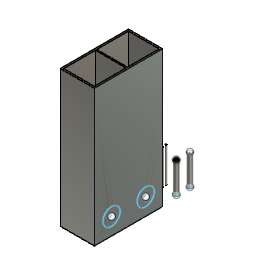
feeder v1 (Autodesk Fusion 360 design; units mm, degrees)
Autodesk Fusion 360 part; units mm, degrees
sketch "Sketch1" plane through (0, 0, 0) normal (0, 0, 1) x (1, 0, 0)
  line L0 (25, 50) -> (-25, 50)
  line L1 (-25, 50) -> (-25, -50)
  line L2 (-25, -50) -> (25, -50)
  line L3 (25, -50) -> (25, 50)
  line L4 (25, 50) -> (-25, -50) construction
  line L5 (-25, 50) -> (25, -50) construction
  dimension "d1" = 100
  constraint horizontal L0
  constraint perpendicular L0 L1
  constraint parallel L0 L2
  constraint parallel L1 L3
  constraint coincident L4 origin
  constraint coincident L5 origin
  measures "d1" distance of L0.end L1.end
extrude "Extrude1" add sketch "Sketch1" along normal blind 200 makes body 1
sketch "Sketch2" plane through (25, 0, 0) normal (1, 0, 0) x (0, 1, 0)
  line L0 (-50, 0) -> (50, 0)
  line L1 (50, 0) -> (50, 200)
  line L2 (50, 200) -> (-50, 200)
  line L3 (-50, 200) -> (-50, 0)
  circle A0 centre (-25, 25) radius 12.5
  circle A1 centre (25, 25) radius 12.5
  dimension "d4" = 25
  dimension "d5" = 25
  measures "d4" diameter of A0
  measures "d5" diameter of A1
extrude "Extrude2" cut sketch "Sketch2" against normal blind 280 contours A1 bodies 1
extrude "Extrude3" cut sketch "Sketch2" against normal blind 155 contours A0 bodies 1
sketch "Sketch3" plane through (0, 0, 200) normal (0, 0, 1) x (-1, 0, 0)
  line L0 (-25, 50) -> (-25, -50)
  line L1 (-25, -50) -> (25, -50)
  line L2 (25, -50) -> (25, 50)
  line L3 (25, 50) -> (-25, 50)
  line L4 (22.5, -47.5) -> (-22.5, -47.5)
  line L5 (-22.5, -47.5) -> (-22.5, 47.5)
  line L6 (-22.5, 47.5) -> (22.5, 47.5)
  line L7 (22.5, 47.5) -> (22.5, -47.5)
  constraint horizontal L4
  constraint vertical L5
  constraint horizontal L6
  constraint vertical L7
extrude "Extrude4" cut sketch "Sketch3" against normal blind 195 contours L4 L5 L6 L7 bodies 1
sketch "Sketch4" plane through (0, 0, 200) normal (0, 0, 1) x (-1, 0, 0)
  line L0 (-22.5, -47.5) -> (-22.5, 47.5)
  line L1 (-22.5, 47.5) -> (22.5, 47.5)
  line L2 (22.5, 47.5) -> (22.5, -47.5)
  line L3 (22.5, -47.5) -> (-22.5, -47.5)
  line L4 (-25, 50) -> (-25, -50)
  line L5 (-25, -50) -> (25, -50)
  line L6 (25, -50) -> (25, 50)
  line L7 (25, 50) -> (-25, 50)
  line L8 (22.5, -1) -> (-22.5, -1)
  line L9 (-22.5, -1) -> (-22.5, 1)
  line L10 (-22.5, 1) -> (22.5, 1)
  line L11 (22.5, 1) -> (22.5, -1)
  constraint horizontal L8
  constraint vertical L9
  constraint horizontal L10
  constraint vertical L11
  constraint coincident L0 L9.end
  constraint coincident L2 L8.start
extrude "Extrude5" add sketch "Sketch4" against normal blind 195 contours L0 L2 L8 L9 L10 L11 bodies 1
sketch "Sketch5" plane through (0, 0, 200) normal (0, 0, 1) x (-1, 0, 0)
  line L0 (-22.5, 1) -> (-22.5, 47.5)
  line L1 (-22.5, 47.5) -> (22.5, 47.5)
  line L2 (22.5, 47.5) -> (22.5, 1)
  line L3 (22.5, 1) -> (-22.5, 1)
  line L4 (-22.5, -1) -> (22.5, -1)
  line L5 (22.5, -1) -> (22.5, -47.5)
  line L6 (22.5, -47.5) -> (-22.5, -47.5)
  line L7 (-22.5, -47.5) -> (-22.5, -1)
  line L8 (-25, 50) -> (-25, -50)
  line L9 (-25, -50) -> (25, -50)
  line L10 (25, -50) -> (25, 50)
  line L11 (25, 50) -> (-25, 50)
extrude "Extrude6" add sketch "Sketch2" against normal blind 2.5 contours A0 bodies 1
extrude "Extrude7" add sketch "Sketch2" against normal blind 2.5 contours A1 bodies 1
sketch "Sketch6" plane through (25, 0, 0) normal (1, 0, 0) x (0, 1, 0)
  circle A0 centre (-25, 25) radius 1.25
  circle A1 centre (25, 25) radius 1.25
  dimension "d18" = 2.5
  dimension "d19" = 2.5
  measures "d18" diameter of A0
  measures "d19" diameter of A1
extrude "Extrude8" cut sketch "Sketch6" against normal blind 5 contours A0 bodies 1
extrude "Extrude9" cut sketch "Sketch6" against normal blind 4 contours A1 bodies 1
sketch "Sketch7" plane through (0, 0, 0) normal (0, 0, 1) x (1, 0, 0)
  circle A0 centre (0, 75) radius 1.2
  dimension "d24" = 2.4
  measures "d24" diameter of A0
extrude "Extrude10" add sketch "Sketch7" along normal blind 51 separate body makes body 2
sketch "Sketch8" plane through (0, 0, 0) normal (0, 0, 1) x (1, 0, 0)
  circle A0 centre (0, 80) radius 1.2
  dimension "d27" = 2.4
  measures "d27" diameter of A0
extrude "Extrude11" add sketch "Sketch8" along normal blind 51 separate body makes body 3
sketch "Sketch9" plane through (0, 0, 0) normal (0, 0, 1) x (1, 0, 0)
  circle A0 centre (20, 75) radius 3.5
  circle A1 centre (20, 95) radius 3.5
  dimension "d30" = 7
  dimension "d31" = 7
  measures "d30" diameter of A0
  measures "d31" diameter of A1
extrude "Extrude12" add sketch "Sketch9" along normal blind 44 separate body contours A1 makes body 4
extrude "Extrude13" add sketch "Sketch9" along normal blind 44 separate body contours A0 makes body 5
sketch "Sketch10" plane through (0, 0, 44) normal (0, 0, 1) x (-1, 0, 0)
  circle A0 centre (-20, -75) radius 3.5
  circle A1 centre (-20, -75) radius 1.25
  circle A2 centre (-20, -95) radius 1.25
  dimension "d36" = 2.5
  dimension "d37" = 2.5
  constraint concentric A0 A1
  measures "d36" diameter of A1
  measures "d37" diameter of A2
extrude "Extrude14" cut sketch "Sketch10" against normal blind 102222222 contours A1 bodies 5
extrude "Extrude15" cut sketch "Sketch10" against normal blind 100 contours A2 bodies 4
